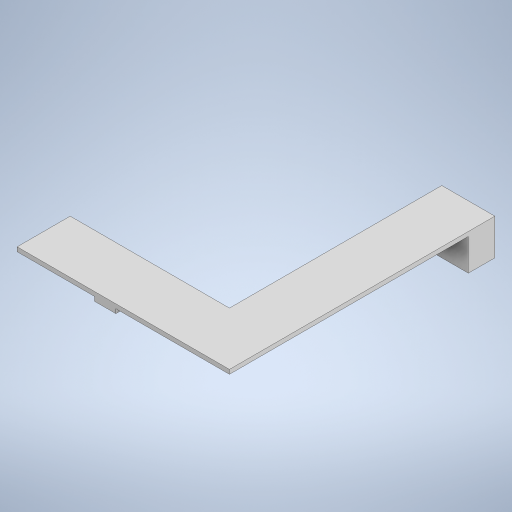
# Autodesk Inventor part: mlx_holder
Saved by Autodesk Inventor 2023 (Build 270158000, 158)
## iProperties
Created: 2023-10-27
Part Number: mlx_holder
Material: Generic
Document SubType Name: Modeling
Designer: mark
Density: 1 g/cm^3
Appearance: Default
Author: mark
Autodesk Inventor part; units mm, degrees
ref_plane "YZ Plane" through (0, 0, 0) normal (1, 0, 0) x (0, 1, 0)
ref_plane "XZ Plane" through (0, 0, 0) normal (0, 1, 0) x (-1, 0, 0)
ref_plane "XY Plane" through (0, 0, 0) normal (0, 0, 1) x (1, 0, 0)
sketch "Sketch1" plane through (0, 0, 0) normal (0, 1, 0) x (-1, 0, 0)
  line L0 (0, 0) -> (-100, 0)
  line L1 (-100, 0) -> (-100, -25)
  line L2 (-100, -25) -> (0, -25)
  line L3 (0, -25) -> (0, 0)
  line L4 (-100, -25) -> (-75, -25)
  line L5 (-75, -25) -> (-75, -125)
  line L6 (-75, -125) -> (-100, -125)
  line L7 (-100, -125) -> (-100, -25)
  dimension "d0" = 100
  dimension "d1" = 25
  dimension "d2" = 25
  dimension "d3" = 100
  constraints: 16 end point, 4 parallel, 2 horizontal, 2 perpendicular
  measures "d0" distance of L2.end L1.end
  measures "d1" distance of L1.end L0.end
  measures "d2" distance of L5.end L6.end
  measures "d3" distance of L6.end L1.end
extrude "Extrusion1" add sketch "Sketch1" along normal blind 2
sketch "Sketch2" plane through (0, 0, 0) normal (0, -1, 0) x (1, 0, 0)
  line L0 (100, 0) -> (100, -125) projected
  line L1 (75, -125) -> (75, -25) projected
  line L2 (100, -125) -> (75, -125)
  line L3 (75, -125) -> (75, -112.5)
  line L4 (75, -112.5) -> (100, -112.5)
  line L5 (100, -112.5) -> (100, -125)
  line L6 (88.5, -112.5) -> (86.5, -112.5)
  line L7 (86.5, -112.5) -> (86.5, -11.5)
  line L8 (86.5, -11.5) -> (88.5, -11.5)
  line L9 (88.5, -11.5) -> (88.5, -112.5)
  line L10 (86.5, -11.5) -> (46.5, -11.5)
  line L11 (46.5, -11.5) -> (46.5, -13.5)
  line L12 (46.5, -13.5) -> (86.5, -13.5)
  line L13 (86.5, -13.5) -> (86.5, -11.5)
  line L14 (0, 0) -> (100, 0) projected
  line L15 (75, -25) -> (0, -25) projected
  line L16 (46.5, 0) -> (36.5, 0)
  line L17 (36.5, 0) -> (36.5, -25)
  line L18 (36.5, -25) -> (46.5, -25)
  line L19 (46.5, -25) -> (46.5, 0)
  dimension "d6" = 12.5
  dimension "d7" = 101
  dimension "d8" = 2
  dimension "d9" = 11.5
  dimension "d10" = 40
  dimension "d11" = 2
  dimension "d12" = 10
  constraints: 32 end point, 8 parallel, 4 horizontal, 4 perpendicular, 4 point on line
  measures "d6" distance of L2.end L3.end
  measures "d7" distance of L6.end L7.end
  measures "d8" distance of L7.end L8.end
  measures "d9" distance between parallel lines of L0 L9
  measures "d10" distance of L12.end L11.end
  measures "d11" distance of L11.end L10.end
  measures "d12" distance of L18.end L17.end
extrude "Extrusion2" add sketch "Sketch2" along normal blind 4 contours L19 L11 L15 L17 L14 | L4 L7 L8 L9 | L10 L7 L12 L11
extrude "Extrusion3" add sketch "Sketch2" along normal blind 15 contours L0 L2 L1 L4
sketch "Sketch3" plane through (0, -15, 0) normal (0, -1, 0) x (1, 0, 0)
  circle A0 centre (90.65, -122.4) radius 1.55
  circle A1 centre (84.35, -122.4) radius 1.55
  line L0 (75, -125) -> (100, -125) projected
  line L1 (75, -112.5) -> (75, -125) projected
  point P0 (0, 0)
  dimension "d17" = 3.1
  dimension "d18" = 3.1
  dimension "d19" = 2.6
  dimension "d20" = 2.6
  dimension "d21" = 6.3
  dimension "d22" = 9.35
  constraints: 2 centre point
  measures "d17" diameter of A0
  measures "d18" diameter of A1
  measures "d19" distance from line of L0 A0.centre
  measures "d20" distance from line of L0 A1.centre
  measures "d21" distance of A1.centre A0.centre
  measures "d22" distance from line of L1 A1.centre
extrude "Extrusion4" add sketch "Sketch3" along normal blind 3
sketch "Sketch4" plane through (0, -4, 0) normal (0, -1, 0) x (1, 0, 0)
  line L0 (46.5, -11.5) -> (46.5, 0) projected
  line L1 (36.5, -25) -> (36.5, 0) projected
  line L2 (46.5, 0) -> (36.5, 0)
  line L3 (36.5, 0) -> (36.5, -6)
  line L4 (36.5, -6) -> (46.5, -6)
  line L5 (46.5, -6) -> (46.5, 0)
  line L6 (46.5, -13.5) -> (46.5, -25) projected
  line L7 (46.5, -25) -> (36.5, -25)
  line L8 (36.5, -25) -> (36.5, -19)
  line L9 (36.5, -19) -> (46.5, -19)
  line L10 (46.5, -19) -> (46.5, -25)
  point P0 (0, 0)
  point P1 (41.5, 0)
  dimension "d25" = 6
  dimension "d26" = 6
  constraints: 16 end point, 4 parallel, 2 horizontal, 2 perpendicular, 2 point on line, 1 midpoint
  measures "d25" distance from line of point (41.5, 0) L4
  measures "d26" distance of L7.end L8.end
extrude "Extrusion5" cut sketch "Sketch4" against normal blind 2
sketch "Sketch5" plane through (86.5, -4, -13.5) normal (-1, 0, 0) x (0, 0, 1)
  line L0 (-99, 4) -> (-11.5, 4) projected
  line L1 (-25.7317, 4) -> (-30.7317, 4)
  line L2 (-30.7317, 4) -> (-30.7317, 2.5)
  line L3 (-30.7317, 2.5) -> (-25.7317, 2.5)
  line L4 (-25.7317, 2.5) -> (-25.7317, 4)
  point P0 (13.5, 4)
  dimension "d29" = 5
  dimension "d30" = 1.5
  constraints: 8 end point, 2 parallel, 1 horizontal, 1 perpendicular, 1 point on line
  measures "d29" distance of L3.end L2.end
  measures "d30" distance of L2.end L1.end
extrude "Extrusion6" cut sketch "Sketch5" against normal blind 2
sketch "Sketch6" plane through (86.5, 0, -13.5) normal (0, 0, -1) x (-1, 0, 0)
  line L0 (11.5, 0) -> (40, 0) projected
  line L1 (21.6385, 0) -> (16.6385, 0)
  line L2 (16.6385, 0) -> (16.6385, -1.5)
  line L3 (16.6385, -1.5) -> (21.6385, -1.5)
  line L4 (21.6385, -1.5) -> (21.6385, 0)
  point P0 (86.5, 0)
  point P1 (16.6385, 0)
  dimension "d33" = 5
  dimension "d34" = 1.5
  constraints: 8 end point, 2 parallel, 1 horizontal, 1 perpendicular, 1 point on line
  measures "d33" distance of L3.end L2.end
  measures "d34" distance of L2.end L1.end
extrude "Extrusion7" cut sketch "Sketch6" against normal blind 2
equation "\"d20\" = d19"
body "Solid1"
